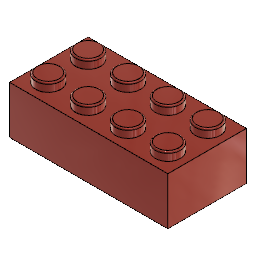
model-Lego-brick (Autodesk Fusion 360 design; units mm, degrees)
Autodesk Fusion 360 part; units mm, degrees
sketch "Sketch1" plane through (0, 0, 0) normal (0, 0, 1) x (1, 0, 0) in component "lego brick"
  line L0 (0, 0) -> (31.8, 0)
  line L1 (31.8, 0) -> (31.8, 15.8)
  line L2 (31.8, 15.8) -> (0, 15.8)
  line L3 (0, 15.8) -> (0, 0)
  dimension "d1" = 31.8
  dimension "d2" = 15.8
  constraint horizontal L0
  constraint vertical L1
  constraint horizontal L2
  constraint vertical L3
  constraint coincident L0.start L3.end
  measures "d1" distance of L0.start L0.end
  measures "d2" distance of L0.start L2.end
extrude "Extrude1" add sketch "Sketch1" along normal blind 9.6 in component "lego brick"
sketch "Sketch1 (2)" plane through (0, 0, 9.6) normal (0, 0, 1) x (-1, 0, 0)
  line L0 (0, -15.8) -> (0, 0)
  line L1 (0, 0) -> (-31.8, 0)
  line L2 (-31.8, 0) -> (-31.8, -15.8)
  line L3 (-31.8, -15.8) -> (0, -15.8)
  circle A0 centre (-3.9, -11.9) radius 2.5
  dimension "d5" = 5
  dimension "d6" = 3.9
  dimension "d7" = 3.9
  measures "d5" diameter of A0
  measures "d6" distance of L3 A0.centre
  measures "d7" distance of L0 A0.centre
extrude "Extrude2" add sketch "Sketch1 (2)" along normal blind 1.7 contours A0 in component "lego brick"
pattern_linear "R-Pattern1" count 4 spacing 8 along (1, 0, 0) count 2 spacing 8 along (0, -1, 0) of "Extrude2" in component "lego brick"
shell "Shell1" thickness 1.7 removed faces 1 at (21.2, 5.2667, 0) in component "lego brick"
sketch "Sketch2" plane through (0, 0, 7.9) normal (0, 0, -1) x (1, 0, 0)
  circle A0 centre (27.9, -3.9) radius 0.8
  circle A1 centre (19.9, -3.9) radius 0.8
  circle A2 centre (11.9, -3.9) radius 0.8
  circle A3 centre (3.9, -3.9) radius 0.8
  circle A4 centre (27.9, -11.9) radius 0.8
  circle A5 centre (19.9, -11.9) radius 0.8
  circle A6 centre (11.9, -11.9) radius 0.8
  circle A7 centre (3.9, -11.9) radius 0.8
  line L0 (1.7, -1.7) -> (1.7, -14.1)
  line L1 (1.7, -14.1) -> (30.1, -14.1)
  line L2 (30.1, -14.1) -> (30.1, -1.7)
  line L3 (30.1, -1.7) -> (1.7, -1.7)
  circle A8 centre (7.9, -7.9) radius 3
  circle A9 centre (7.9, -7.9) radius 2
  dimension "d15" = 6
  dimension "d16" = -1
  measures "d15" diameter of A8
extrude "Extrude3" add sketch "Sketch2" along normal blind 7 contours A8 in component "lego brick"
pattern_linear "R-Pattern2" count 3 spacing 8 along (1, 0, 0) of "Extrude3" in component "lego brick"
fillet "Fillet1" radius 0.3 8 edges at (30.2308, 12.804, 11.3) (22.2308, 12.804, 11.3) (14.2308, 12.804, 11.3) (6.2308, 12.804, 11.3) (6.2308, 4.804, 11.3) (14.2308, 4.804, 11.3) (22.2308, 4.804, 11.3) (30.2308, 4.804, 11.3) in component "lego brick"
fillet "Fillet2" radius 0.3 3 edges at (13.103, 8.9848, 0.9) (21.103, 8.9848, 0.9) (5.103, 8.9848, 0.9) in component "lego brick"
component "lego brick" placed x (1, 0, 0) y (0, 1, 0) z (0, 0, 1) at (0, 0, 0)
